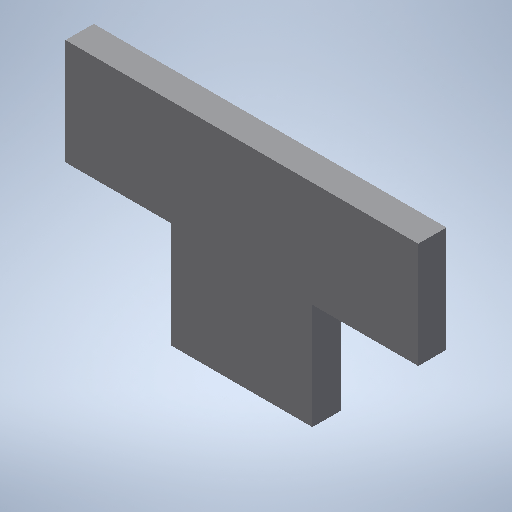
# Autodesk Inventor part: Seguro
Saved by Autodesk Inventor 2025 (Build 290162000, 162)
## iProperties
Created: 2024-10-23
Part Number: Seguro
Material: Generic
Document SubType Name: Modeling
Designer: feder
Density: 1 g/cm^3
Appearance: Default
Author: feder
Autodesk Inventor part; units mm, degrees
ref_plane "YZ Plane" through (0, 0, 0) normal (1, 0, 0) x (0, 1, 0)
ref_plane "XZ Plane" through (0, 0, 0) normal (0, 1, 0) x (-1, 0, 0)
ref_plane "XY Plane" through (0, 0, 0) normal (0, 0, 1) x (1, 0, 0)
sketch "Sketch1" plane through (0, 0, 0) normal (0, 0, 1) x (1, 0, 0)
  line L0 (10, 0) -> (-10, 0)
  line L1 (-10, 0) -> (-10, 15)
  line L2 (-10, 15) -> (10, 15)
  line L3 (10, 15) -> (10, 0)
  line L4 (25, 15) -> (-25, 15)
  line L5 (-25, 15) -> (-25, 30)
  line L6 (-25, 30) -> (25, 30)
  line L7 (25, 30) -> (25, 15)
  point P0 (0, 0)
  point P1 (0, 0)
  point P2 (0, 15)
  point P3 (0, 15)
  point P4 (10, 15)
  dimension "d0" = 20
  dimension "d1" = 15
  dimension "d2" = 15
  dimension "d3" = 50
  constraints: 16 end point, 4 parallel, 3 coincident, 3 midpoint, 2 horizontal, 2 perpendicular, 1 vertical alignment
  measures "d0" distance of L0.start L0.end
  measures "d1" distance of L2.end L0.start
  measures "d2" distance of L4.end L5.end
  measures "d3" distance of L4.start L4.end
extrude "Extrusion1" add sketch "Sketch1" along normal blind 4
body "Solid1"
